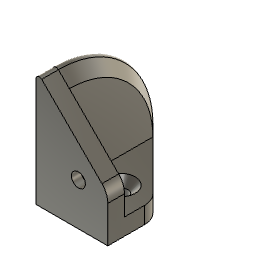
Door_Stop (Autodesk Fusion 360 design; units mm, degrees)
Autodesk Fusion 360 part; units mm, degrees
note: some values were not read from the file. Chosen so that the rebuilt part matches the saved one: which face or edge a step refers to; which pieces of a blend or face edit are solid. Set by a fixed rule: which sketch regions a step uses.
sketch "Skizze1" plane through (0, 0, 0) normal (0, 0, 1) x (1, 0, 0)
  line L0 (0, 0) -> (0, 35)
  line L1 (0, 0) -> (21.5, 0)
  line L2 (0, 35) -> (33.3017, 35) construction
  line L3 (21.5, 0) -> (21.5, 13.5)
  line L4 (21.5, 13.5) -> (0, 35)
  dimension "d1" = 35
  dimension "d2" = 21.5
  constraint coincident L0.start L1.start
  constraint vertical L0
  constraint perpendicular L0 L1
  constraint horizontal L2
  constraint perpendicular L1 L3
  measures "d1" distance of L0.start L0.end
  measures "d2" distance of L0.start L1.end
sketch "Skizze2" plane through (0, 0, 0) normal (0, 1, 0) x (1, 0, 0)
  line L0 (0, 0) -> (0, -35)
  line L1 (0, 0) -> (21.5, 0)
  line L2 (0, -35) -> (37.4833, -35) construction
  line L3 (21.5, 0) -> (21.5, -13.5)
  line L4 (0, -35) -> (21.5, -13.5)
  dimension "d4" = 35
  dimension "d5" = 21.5
  constraint coincident L0.start L1.start
  constraint perpendicular L0 L1
  constraint horizontal L2
  constraint perpendicular L1 L3
  measures "d4" distance of L0.end L0.start
  measures "d5" distance of L0.start L1.end
extrude "Extrusion1" add sketch "Skizze1" along normal blind 5
extrude "Extrusion2" add sketch "Skizze2" along normal blind 5
sketch "Skizze4" plane through (0, 0, 0) normal (1, 0, 0) x (0, 1, 0)
  arc A0 (35, 5) -> (5, 35) centre (5, 5) ccw
  line L0 (5, 35) -> (5, 5)
  line L1 (5, 5) -> (35, 5)
  point P0 (5, 5)
  point P1 (35, 5)
  point P2 (5, 35)
  constraint coincident P2 A0.end
  constraint coincident P1 A0.start
  constraint coincident P0 A0.centre
  constraint perpendicular L0 L1
extrude "Extrusion4" add sketch "Skizze4" along normal blind 5
chamfer "Fase1" distance 5 distance2 5 1 edges at (5, 26.2132, 26.2132) measured on face at (5, 10.4064, 21.7459)
sketch "Skizze5" plane through (0, 0, 5) normal (0, 0, 1) x (-1, 0, 0)
  line L0 (-5, -30) -> (-5, -5)
  line L1 (-5, -5) -> (-21.5, -5)
  line L2 (-21.5, -5) -> (-21.5, -13.5)
  line L3 (-21.5, -13.5) -> (-5, -30)
  line L4 (-5, -5) -> (-12.7, -5)
  line L5 (-12.7, -5) -> (-12.7, -12.7)
  line L6 (-12.7, -12.7) -> (-5, -12.7)
  line L7 (-5, -12.7) -> (-5, -5)
  dimension "d19" = 7.7
  dimension "d20" = 7.7
  constraint horizontal L4
  constraint vertical L5
  constraint horizontal L6
  constraint vertical L7
  constraint coincident L0.end L1.start
  measures "d19" distance of L0.end L4.end
  measures "d20" distance of L0.end L6.end
sketch "Skizze6" plane through (0, 5, 0) normal (0, 1, 0) x (-1, 0, 0)
  line L0 (-5, 5) -> (-5, 30)
  line L1 (-5, 30) -> (-21.5, 13.5)
  line L2 (-21.5, 13.5) -> (-21.5, 5)
  line L3 (-21.5, 5) -> (-5, 5)
  line L4 (-5, 5) -> (-12.7, 5)
  line L5 (-12.7, 5) -> (-12.7, 12.7)
  line L6 (-12.7, 12.7) -> (-5, 12.7)
  line L7 (-5, 12.7) -> (-5, 5)
  dimension "d21" = 7.7
  dimension "d22" = 7.7
  constraint horizontal L4
  constraint vertical L5
  constraint horizontal L6
  constraint vertical L7
  constraint coincident L0.start L3.end
  measures "d21" distance of L0.start L4.end
  measures "d22" distance of L0.start L6.end
hole "Bohrung1" at (12.7, 12.7, 5) direction (0, 0, -1) diameter 4.2 depth 13 tip angle 180 countersink diameter 8.6 countersink angle 90
hole "Bohrung2" at (12.7, 5, 12.7) direction (0, -1, 0) diameter 4.2 depth 13 tip angle 180 countersink diameter 8.6 countersink angle 90
fillet "Abrundung1" radius 1 6 edges at (0.0005, 35, 5) (0.001, 26.2132, 26.2132) (0, 26.2132, 26.2132) (0.0005, 5, 35) (0, 35, 2.5) (0, 2.5, 35)
fillet "Abrundung2" radius 6 1 edges at (21.5, 2.5, 13.5)
fillet "Abrundung3" radius 6 1 edges at (21.5, 13.5, 2.5)
